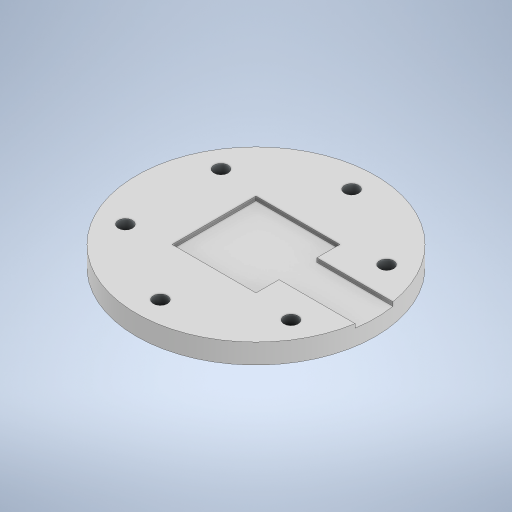
# Autodesk Inventor part: Base1
Saved by Autodesk Inventor 2023 (Build 270158000, 158)
## iProperties
Created: 2023-02-08
Part Number: Base1
Material: Ogólny
Document SubType Name: Modeling
Designer: kamil
Density: 1 g/cm^3
Appearance: Domyślna
Author: kamil
Autodesk Inventor part; units mm, degrees
ref_plane "YZ Plane" through (0, 0, 0) normal (1, 0, 0) x (0, 1, 0)
ref_plane "XZ Plane" through (0, 0, 0) normal (0, 1, 0) x (-1, 0, 0)
ref_plane "XY Plane" through (0, 0, 0) normal (0, 0, 1) x (1, 0, 0)
sketch "Szkic1" plane through (0, 0, 0) normal (0, 1, 0) x (-1, 0, 0)
  circle A0 centre (0, 0) radius 60
  dimension "d0" = 120
  constraints: 2 coincident, 1 centre point
  measures "d0" diameter of A0
extrude "Wyciągnięcie proste1" add sketch "Szkic1" along normal blind 10
sketch "Szkic2" plane through (0, 10, 0) normal (0, 1, 0) x (1, 0, 0)
  circle A0 centre (0, 48) radius 3.55
  circle A1 centre (-41.5692, 24) radius 3.55
  circle A2 centre (-41.5692, -24) radius 3.55
  circle A3 centre (0, -48) radius 3.55
  circle A4 centre (41.5692, -24) radius 3.55
  circle A5 centre (41.5692, 24) radius 3.55
  point P0 (0, 0)
  dimension "d13" = 7.1
  dimension "d16" = 360
  dimension "d20" = 48
  constraints: 6 centre point, 13 other
  measures "d13" diameter of A0
  measures "d20" distance of A0.centre point (0, 0)
extrude "Wyciągnięcie proste2" cut sketch "Szkic2" against normal blind 5
sketch "Szkic3" plane through (0, 10, 0) normal (0, 1, 0) x (1, 0, 0)
  line L0 (-21.05, -21.05) -> (21.05, -21.05)
  line L1 (21.05, -21.05) -> (21.05, 21.05)
  line L2 (21.05, 21.05) -> (-21.05, 21.05)
  line L3 (-21.05, 21.05) -> (-21.05, -21.05)
  line L4 (-21.05, -21.05) -> (21.05, 21.05)
  line L5 (-21.05, 21.05) -> (21.05, -21.05)
  point P0 (0, 0)
  point P1 (0, 0)
  dimension "d21" = 42.1
  dimension "d22" = 42.1
  constraints: 12 end point, 2 parallel, 1 coincident, 1 horizontal, 1 midpoint, 1 perpendicular
  measures "d21" distance of L1.end L2.end
  measures "d22" distance of L2.end L0.start
extrude "Wyciągnięcie proste3" cut sketch "Szkic3" against normal blind 2
sketch "Szkic4" plane through (0, 10, 0) normal (0, 1, 0) x (1, 0, 0)
  line L0 (21.05, 21.05) -> (21.05, -21.05) projected
  line L1 (21.05, -9.5) -> (61.05, -9.5)
  line L2 (61.05, -9.5) -> (61.05, 9.5)
  line L3 (61.05, 9.5) -> (21.05, 9.5)
  line L4 (21.05, 9.5) -> (21.05, -9.5)
  point P0 (0, 0)
  point P1 (21.05, 0)
  dimension "d25" = 19
  dimension "d26" = 40
  constraints: 8 end point, 2 midpoint, 2 parallel, 1 horizontal, 1 perpendicular, 1 point on line
  measures "d25" distance of L2.end L1.end
  measures "d26" distance of L2.end L3.end
extrude "Wyciągnięcie proste4" cut sketch "Szkic4" against normal blind 2
